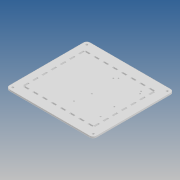
# Autodesk Inventor part: 000.101 - Bottom
Saved by Autodesk Inventor 2020 (Build 240168000, 168)
## iProperties
Created: 2021-06-27
Part Number: 000.101 - Bottom
Material: Типовые
Document SubType Name: Modeling
Designer: Петров Иван
Mass: 97.1844 g
Surface Area: 696.432 cm^2
Volume: 97.1844 cm^3
Density: 1 g/cm^3
Appearance: По умолчанию
Author: Петров Иван
Autodesk Inventor part; units mm, degrees
ref_plane "YZ Plane" through (0, 0, 0) normal (1, 0, 0) x (0, 1, 0)
ref_plane "XZ Plane" through (0, 0, 0) normal (0, 1, 0) x (-1, 0, 0)
ref_plane "XY Plane" through (0, 0, 0) normal (0, 0, 1) x (1, 0, 0)
sketch "Эскиз1" plane through (0, 0, 0) normal (0, 1, 0) x (-1, 0, 0)
  line L0 (-87.5, 80.5) -> (87.5, 80.5) construction
  line L1 (87.5, 80.5) -> (87.5, -80.5) construction
  line L2 (87.5, -80.5) -> (-87.5, -80.5) construction
  line L3 (-87.5, -80.5) -> (-87.5, 80.5) construction
  line L4 (-87.5, 80.5) -> (87.5, -80.5) construction
  line L5 (87.5, 80.5) -> (-87.5, -80.5) construction
  circle A0 centre (87.5, 80.5) radius 2
  circle A1 centre (87.5, -80.5) radius 2
  circle A2 centre (-87.5, 80.5) radius 2
  circle A3 centre (-87.5, -80.5) radius 2
  arc A4 (87.5, 73) -> (80, 80.5) centre (87.5, 80.5) ccw
  arc A5 (80, -80.5) -> (87.5, -73) centre (87.5, -80.5) ccw
  arc A6 (-87.5, -73) -> (-80, -80.5) centre (-87.5, -80.5) ccw
  arc A7 (-80, 80.5) -> (-87.5, 73) centre (-87.5, 80.5) ccw
  line L6 (87.5, 73) -> (87.5, -73)
  line L7 (80, 80.5) -> (-80, 80.5)
  line L8 (-87.5, 73) -> (-87.5, -73)
  line L9 (-80, -80.5) -> (80, -80.5)
  line L10 (87.5, 88) -> (-87.5, 88)
  line L11 (-95, 80.5) -> (-95, -80.5)
  line L12 (87.5, -88) -> (-87.5, -88)
  line L13 (95, 80.5) -> (95, -80.5)
  point P0 (0, 0)
  dimension "d0" = 175
  dimension "d1" = 161
  dimension "d2" = 4
  dimension "d3" = 4
  dimension "d4" = 4
  dimension "d5" = 4
  dimension "d6" = 15
  dimension "d7" = 15
  dimension "d8" = 15
  dimension "d9" = 15
  constraints: 28 end point, 16 point on circle, 8 centre point, 8 coincident, 7 point on line, 5 tangent, 2 horizontal, 2 midpoint, 2 parallel, 1 perpendicular
  measures "d0" distance of L1.end L2.end
  measures "d1" distance of L0.end L1.end
  measures "d2" diameter of A0
  measures "d3" diameter of A1
  measures "d4" diameter of A2
  measures "d5" diameter of A3
  measures "d6" diameter of A4
  measures "d7" diameter of A5
  measures "d8" diameter of A6
  measures "d9" diameter of A7
extrude "Выдавливание1" add sketch "Эскиз1" along normal blind 3
sketch "Эскиз3" plane through (0, 3, 0) normal (0, 1, 0) x (1, 0, 0)
  line L0 (-80, -65) -> (-77, -65)
  line L1 (-77, -65) -> (-77, -55)
  line L2 (-77, -55) -> (-80, -55)
  line L3 (-80, -55) -> (-80, -65)
  line L4 (-87.5, -88) -> (87.5, -88) projected
  line L5 (-95, 80.5) -> (-95, -80.5) projected
  point P0 (0, 0)
  dimension "d16" = 3
  dimension "d17" = 10
  dimension "d18" = 23
  dimension "d49" = 15
  constraints: 8 end point, 2 parallel, 1 horizontal, 1 perpendicular
  measures "d16" distance of L2.end L1.end
  measures "d17" distance of L1.end L0.end
  measures "d18" distance between parallel lines of L4 L0
  measures "d49" distance between parallel lines of L5 L3
extrude "Выдавливание3" cut sketch "Эскиз3" against normal blind 3
pattern_linear "Прямоуг.массив1" count 7 spacing 20 along (0, 0, -1) of "Выдавливание3"
sketch "Эскиз4" plane through (0, 3, 0) normal (0, 1, 0) x (1, 0, 0)
  line L0 (-77, -65) -> (-77, -55) projected
  line L1 (-77, -65) -> (-67, -65)
  line L2 (-67, -65) -> (-67, -68)
  line L3 (-67, -68) -> (-77, -68)
  line L4 (-77, -68) -> (-77, -65)
  point P0 (0, 0)
  dimension "d24" = 10
  dimension "d25" = 3
  constraints: 8 end point, 2 parallel, 1 horizontal, 1 perpendicular
  measures "d24" distance of L2.end L3.end
  measures "d25" distance of L1.end L2.end
extrude "Выдавливание4" cut sketch "Эскиз4" against normal blind 3
pattern_linear "Прямоуг.массив2" count 8 spacing 20 along (1, 0, 0) of "Выдавливание4"
sketch "Эскиз5" plane through (0, 3, 0) normal (0, 1, 0) x (1, 0, 0)
  line L0 (73, -65) -> (76, -65)
  line L1 (76, -65) -> (76, -55)
  line L2 (76, -55) -> (73, -55)
  line L3 (73, -55) -> (73, -65)
  point P0 (0, 0)
  dimension "d31" = 3
  dimension "d32" = 10
  constraints: 8 end point, 2 parallel, 1 coincident, 1 horizontal, 1 perpendicular
  measures "d31" distance of L2.end L1.end
  measures "d32" distance of L1.end L0.end
extrude "Выдавливание5" cut sketch "Эскиз5" against normal blind 3
pattern_linear "Прямоуг.массив3" count 7 spacing 20 along (0, 0, -1) of "Выдавливание5"
sketch "Эскиз6" plane through (0, 3, 0) normal (0, 1, 0) x (1, 0, 0)
  line L0 (-77, 55) -> (-77, 65) projected
  line L1 (-77, 65) -> (-67, 65)
  line L2 (-67, 65) -> (-67, 68)
  line L3 (-67, 68) -> (-77, 68)
  line L4 (-77, 68) -> (-77, 65)
  point P0 (0, 0)
  dimension "d38" = 10
  dimension "d39" = 3
  constraints: 8 end point, 2 parallel, 1 horizontal, 1 perpendicular
  measures "d38" distance of L3.end L2.end
  measures "d39" distance of L2.end L1.end
extrude "Выдавливание6" cut sketch "Эскиз6" against normal blind 3
pattern_linear "Прямоуг.массив4" count 8 spacing 20 along (1, 0, 0) of "Выдавливание6"
sketch "Эскиз7" plane through (0, 3, 0) normal (0, 1, 0) x (1, 0, 0)
  circle A0 centre (59.5, 51.5) radius 1.35 projected
  circle A1 centre (10.5, 51.5) radius 1.35 projected
  circle A2 centre (10.5, -6.5) radius 1.35 projected
  circle A3 centre (59.5, -6.5) radius 1.35 projected
  point P0 (0, 0)
extrude "Выдавливание7" cut sketch "Эскиз7" against normal blind 3
sketch "Эскиз8" plane through (0, 3, 0) normal (0, 1, 0) x (1, 0, 0)
  circle A0 centre (63, 46) radius 1.375 projected
  circle A1 centre (63, -40) radius 1.375 projected
  circle A2 centre (5, -40) radius 1.375 projected
  circle A3 centre (5, 46) radius 1.375 projected
  point P0 (0, 0)
extrude "Выдавливание8" cut sketch "Эскиз8" against normal blind 3
